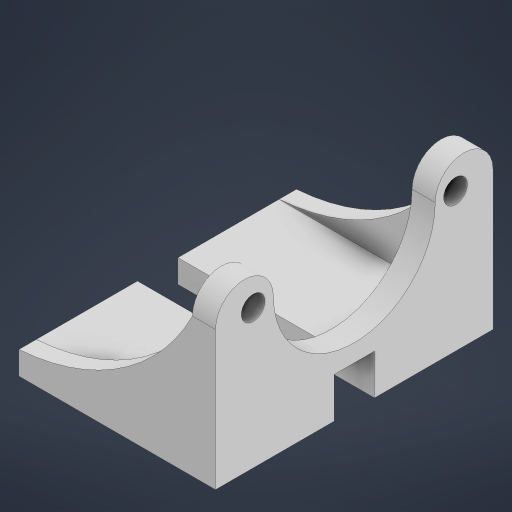
# Autodesk Inventor part: soporte_stepper
Saved by Autodesk Inventor 2023.1 (Build 271208000, 208)
## iProperties
Created: 2022-10-26
Part Number: soporte_stepper
Material: Generic
Document SubType Name: Modeling
Designer: amtat
Density: 1 g/cm^3
Appearance: Default
Author: amtat
Autodesk Inventor part; units mm, degrees
ref_plane "YZ Plane" through (0, 0, 0) normal (1, 0, 0) x (0, 1, 0)
ref_plane "XZ Plane" through (0, 0, 0) normal (0, 1, 0) x (-1, 0, 0)
ref_plane "XY Plane" through (0, 0, 0) normal (0, 0, 1) x (1, 0, 0)
sketch "Sketch1" plane through (0, 0, 0) normal (1, 0, 0) x (0, 1, 0)
  circle A0 centre (0, 0) radius 2.05
  line L0 (0, 0) -> (0, -35)
  circle A1 centre (0, -35) radius 2.05
  line L1 (0, 0) -> (0, -17.5)
  arc A2 (0, -3.5) -> (0, -31.5) centre (0, -17.5) ccw
  arc A3 (0, -31.5) -> (-3.5, -35) centre (0, -35) ccw
  arc A4 (-3.5, 0) -> (0, -3.5) centre (0, 0) ccw
  line L2 (0, 0) -> (-24, 0)
  line L3 (-24, 0) -> (-24, -35)
  line L4 (-24, -35) -> (0, -35)
  line L5 (0, -3.5) -> (0, 6.5)
  line L6 (0, 6.5) -> (0, 1.5)
  arc A5 (-4.7697, 0) -> (0, 6.5) centre (0, 1.5) ccw
  line L7 (0, 6.5) -> (-24, 6.5)
  line L8 (-24, 6.5) -> (-24, 0)
  line L9 (0, -31.5) -> (0, -36.5)
  arc A6 (0, -41.5) -> (-4.7697, -35) centre (0, -36.5) ccw
  line L10 (0, -41.5) -> (-24, -41.5)
  line L11 (-24, -41.5) -> (-24, -35)
  dimension "d0" = 4.1
  dimension "d1" = 35
  dimension "d2" = 4.1
  dimension "d3" = 17.5
  dimension "d4" = 28
  dimension "d5" = 24
  dimension "d6" = 10
  dimension "d7" = 5
  constraints: 24 end point, 12 point on circle, 7 centre point, 7 coincident, 5 point on line, 4 perpendicular, 3 horizontal, 2 midpoint, 2 vertical
  measures "d0" diameter of A0
  measures "d1" distance of L0.start L0.end
  measures "d2" diameter of A1
  measures "d3" distance of L0.start L1.end
  measures "d4" diameter of A2
  measures "d5" distance of L2.start L2.end
  measures "d6" distance of L5.start L5.end
  measures "d7" distance of L9.start L9.end
extrude "Extrusion1" add sketch "Sketch1" along normal blind 4 contours A0 L5 A5 L0 | A0 L2 L8 L7 L5 | L0 A4 L2 A0 | A5 L2 A4 | A2 A6 L4 L3 L2 A5 | A6 L10 L11 L4 A1 L0 | L0 A1 L4 A3 | A3 L4 A6
sketch "Sketch2" plane through (0, 0, 0) normal (-1, 0, 0) x (0, 0, 1)
  line L0 (6.5, 0) -> (6.5, -24) projected
  arc A0 (6.5, 0) -> (-3.5, 0) centre (1.5, 0) ccw projected
  arc A1 (-31.5, 0) -> (-3.5, 0) centre (-17.5, 0) ccw projected
  arc A2 (-31.5, 0) -> (-41.5, 0) centre (-36.5, 0) ccw projected
  line L1 (-41.5, -24) -> (-41.5, 0) projected
  line L2 (6.5, -24) -> (-41.5, -24) projected
  circle A3 centre (0, 0) radius 2.05 projected
  circle A4 centre (-35, 0) radius 2.05 projected
  line L3 (-17.5, 0) -> (-17.5, -24)
  line L4 (-17.5, -24) -> (-14, -24)
  line L5 (6.5, -24) -> (-41.5, -24) projected
  line L6 (-17.5, -24) -> (-21, -24)
  line L7 (-21, -24) -> (-21, -20)
  line L8 (-21, -20) -> (-41.5, -20)
  line L9 (-14, -24) -> (-14, -20)
  line L10 (-14, -20) -> (6.5, -20)
  dimension "d10" = 3.5
  dimension "d11" = 3.5
  dimension "d12" = 4
  constraints: 14 end point, 6 point on line, 3 perpendicular, 1 midpoint
  measures "d10" distance of L3.end L4.end
  measures "d11" distance of L3.end L6.end
  measures "d12" distance of L6.end L7.end
extrude "Extrusion2" add sketch "Sketch2" along normal blind 30 contours L0 L2 L9 L10 | L2 L1 L8 L7
sketch "Sketch3" plane through (0, 0, 0) normal (-1, 0, 0) x (0, 0, 1)
  line L0 (-21, -20) -> (-21, -24) projected
  line L1 (-14, -24) -> (-21, -24) projected
  line L2 (-14, -24) -> (-14, -20) projected
  line L3 (-14, -20) -> (6.5, -20) projected
  line L4 (6.5, 0) -> (6.5, -20) projected
  arc A0 (6.5, 0) -> (-3.5, 0) centre (1.5, 0) ccw projected
  arc A1 (-31.5, 0) -> (-3.5, 0) centre (-17.5, 0) ccw projected
  arc A2 (-31.5, 0) -> (-41.5, 0) centre (-36.5, 0) ccw projected
  line L5 (-41.5, -20) -> (-41.5, 0) projected
  line L6 (-41.5, -20) -> (-21, -20) projected
  circle A3 centre (0, 0) radius 2.05 projected
  circle A4 centre (-35, 0) radius 2.05 projected
  line L7 (-21, -24) -> (-21, -20) projected
  line L8 (-21, -24) -> (-21, -17)
  line L9 (-21, -17) -> (-14, -17)
  line L10 (-14, -17) -> (-14, -24)
  dimension "d15" = 7
  constraints: 6 end point, 2 perpendicular, 1 point on line
  measures "d15" distance of L0.end L8.end
extrude "Extrusion3" cut sketch "Sketch3" against normal blind 30 contours L8 L9 L10 L2 L1 L0
sketch "Sketch4" plane through (4, 0, -41.5) normal (0, 0, -1) x (-1, 0, 0)
  line L0 (4, -20) -> (4, 0) projected
  line L1 (4, 0) -> (0, 0) projected
  line L2 (0, -24) -> (0, 0) projected
  line L3 (34, -24) -> (0, -24) projected
  line L4 (34, -20) -> (34, -24) projected
  line L5 (4, -20) -> (34, -20) projected
  line L6 (4, -20) -> (34, -20) projected
  arc A0 (4, 0) -> (34, -20) centre (36.5962, 16.3943) ccw
  point P0 (4, 0)
  constraints: 2 point on circle, 1 centre point
extrude "Extrusion4" add sketch "Sketch4" against normal blind 3 contours L0 A0 L5
sketch "Sketch5" plane through (0, 0, 6.5) normal (0, 0, 1) x (1, 0, 0)
  line L0 (0, 0) -> (0, -20) projected
  arc A0 (-30, -20) -> (0, 0) centre (-32.5962, 16.3943) ccw projected
  line L1 (0, -20) -> (-30, -20) projected
  point P0 (0, 0)
extrude "Extrusion5" add sketch "Sketch5" against normal blind 3
fillet "Fillet1" radius 3 2 edges at (0, -20, -29.75) (0, -20, -5.25)
body "Solid1"
